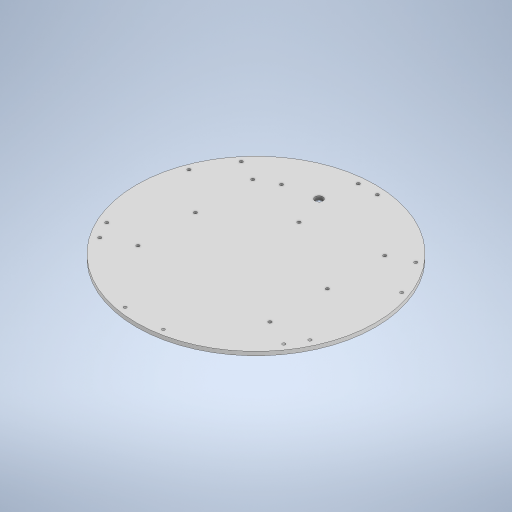
# Autodesk Inventor part: 中間台1
Saved by Autodesk Inventor 2023 (Build 270158000, 158)
## iProperties
Created: 2022-12-03
Part Number: 中間台1
Material: 一般
Document SubType Name: Modeling
Designer: RiSA
Density: 1 g/cm^3
Appearance: 既定
Author: RiSA
Autodesk Inventor part; units mm, degrees
ref_plane "YZ Plane" through (0, 0, 0) normal (1, 0, 0) x (0, 1, 0)
ref_plane "XZ Plane" through (0, 0, 0) normal (0, 1, 0) x (-1, 0, 0)
ref_plane "XY Plane" through (0, 0, 0) normal (0, 0, 1) x (1, 0, 0)
sketch "スケッチ1" plane through (0, 0, 0) normal (0, 1, 0) x (-1, 0, 0)
  circle A0 centre (0, 0) radius 125
  dimension "d0" = 250
  constraints: 1 centre point, 1 coincident
  measures "d0" diameter of A0
extrude "押し出し1" add sketch "スケッチ1" along normal blind 4
sketch "スケッチ2" plane through (0, 4, 0) normal (0, 1, 0) x (1, 0, 0)
  line L0 (75, -84.411) -> (-75, -84.411)
  line L1 (-75, -84.411) -> (-75, 95.589)
  line L2 (-75, 95.589) -> (75, 95.589)
  line L3 (75, 95.589) -> (75, -84.411)
  line L4 (75, -84.411) -> (-75, 95.589) construction
  line L5 (-75, -84.411) -> (75, 95.589) construction
  circle A0 centre (0, 0) radius 121.5
  line L6 (0, 0) -> (0, -125) construction
  circle A1 centre (0, 0) radius 125 projected
  line L7 (0, 0) -> (108.2532, 62.5) construction
  line L8 (0, 0) -> (-108.2532, 62.5) construction
  circle A2 centre (-16.75, 82.589) radius 4.1
  point P0 (0, 5.589)
  dimension "d3" = 150
  dimension "d4" = 180
  dimension "d5" = 243
  dimension "d8" = 360
  dimension "d12" = 16.75
  dimension "d13" = 13
  dimension "d14" = 8.2
  constraints: 18 end point, 2 centre point, 2 coincident, 2 midpoint, 2 parallel, 2 point on circle, 1 horizontal, 1 perpendicular, 1 vertical, 1 vertical alignment, 11 other
  measures "d3" distance of L1.end L2.end
  measures "d4" distance of L0.end L1.end
  measures "d5" diameter of A0
  measures "d12" horizontal distance of point (0, 0) point (-16.75, 82.589)
  measures "d13" distance from line of L2 point (-16.75, 82.589)
  measures "d14" diameter of A2
extrude "押し出し2" cut sketch "スケッチ2" against normal blind 4 contours A2
sketch "スケッチ4" plane through (0, 4, 0) normal (0, 1, 0) x (1, 0, 0)
  circle A0 centre (0, 0) radius 121.5
  line L0 (75, -84.411) -> (-75, -84.411)
  line L1 (-75, -84.411) -> (-75, 95.589)
  line L2 (-75, 95.589) -> (75, 95.589)
  line L3 (75, 95.589) -> (75, -84.411)
  line L4 (75, -84.411) -> (-75, 95.589) construction
  line L5 (-75, -84.411) -> (75, 95.589) construction
  line L6 (0, 0) -> (0, -29.9183)
  point P0 (0, 5.589)
  point P1 (69, -54.411)
  point P2 (69, 5.589)
  point P3 (69, 65.589)
  point P4 (-69, -54.411)
  point P5 (-69, 5.589)
  point P6 (-69, 65.589)
  dimension "d17" = 243
  dimension "d18" = 150
  dimension "d19" = 180
  dimension "d20" = 30
  dimension "d21" = 6
  dimension "d22" = 60
  dimension "d23" = 60
  constraints: 14 end point, 3 symmetric about line, 2 midpoint, 2 parallel, 2 point on circle, 1 centre point, 1 coincident, 1 horizontal, 1 perpendicular, 1 vertical
  measures "d17" diameter of A0
  measures "d18" distance of L1.end L2.end
  measures "d19" distance of L0.end L1.end
  measures "d20" distance from line of L0 point (69, -54.411)
  measures "d21" distance from line of L3 point (69, -54.411)
  measures "d22" distance of point (69, -54.411) point (69, 5.589)
  measures "d23" distance of point (69, 5.589) point (69, 65.589)
hole "穴1" at (69, 4, 54.411) at (69, 4, -5.589) at (69, 4, -65.589) at (-69, 4, -65.589) at (-69, 4, -5.589) at (-69, 4, 54.411) direction (0, -1, 0) diameter 3.2 end through all
sketch "スケッチ5" plane through (0, 4, 0) normal (0, 1, 0) x (1, 0, 0)
  point P0 (0, 0)
  point P1 (0, -116.86)
  point P2 (20, -116.86)
  point P3 (-20, -116.86)
  point P4 (111.2037, 41.1095)
  point P5 (91.2037, 75.7505)
  point P6 (101.2037, 58.43)
  point P7 (-91.2037, 75.7505)
  point P8 (-111.2037, 41.1095)
  point P9 (-101.2037, 58.43)
  dimension "d31" = 116.86
  dimension "d32" = 20
  dimension "d33" = 20
  dimension "d36" = 360
  constraints: 10 other
  measures "d31" distance of point (0, 0) point (0, -116.86)
  measures "d32" distance of point (0, -116.86) point (20, -116.86)
  measures "d33" distance of point (-20, -116.86) point (0, -116.86)
hole "穴2" at (20, 4, 116.86) at (-20, 4, 116.86) at (111.2037, 4, -41.1095) at (91.2037, 4, -75.7505) at (-91.2037, 4, -75.7505) at (-111.2037, 4, -41.1095) direction (0, -1, 0) diameter 3.2 depth 10
sketch "スケッチ6" plane through (0, 4, 0) normal (0, 1, 0) x (1, 0, 0)
  point P0 (0, 0)
  point P1 (0, 116.86)
  point P2 (-10, 116.86)
  point P3 (10, 116.86)
  point P4 (-106.2037, -49.7697)
  point P5 (-96.2037, -67.0903)
  point P6 (-101.2037, -58.43)
  point P7 (96.2037, -67.0903)
  point P8 (106.2037, -49.7697)
  point P9 (101.2037, -58.43)
  dimension "d45" = 116.86
  dimension "d46" = 10
  dimension "d47" = 10
  dimension "d50" = 360
  constraints: 10 other
  measures "d45" distance of point (0, 0) point (0, 116.86)
  measures "d46" distance of point (0, 116.86) point (-10, 116.86)
  measures "d47" distance of point (0, 116.86) point (10, 116.86)
hole "穴3" at (-10, 4, -116.86) at (10, 4, -116.86) at (-106.2037, 4, 49.7697) at (-96.2037, 4, 67.0903) at (96.2037, 4, 67.0903) at (106.2037, 4, 49.7697) direction (0, -1, 0) diameter 3.2 depth 10
sketch "スケッチ7" plane through (0, 4, 0) normal (0, 1, 0) x (1, 0, 0)
  circle A0 centre (-16.75, 82.589) radius 4.1 projected
  line L0 (-16.75, 82.589) -> (-27.75, 63.5364) construction
  line L1 (-16.75, 82.589) -> (5.25, 82.589) construction
  line L2 (-27.75, 63.5364) -> (-49.4006, 76.0364)
  line L3 (-49.4006, 76.0364) -> (-6.0994, 51.0364) construction
  point P0 (0, 0)
  dimension "d59" = 22
  dimension "d60" = 120
  dimension "d61" = 25
  dimension "d62" = 50
  constraints: 8 end point, 2 coincident, 1 equal length, 1 horizontal, 1 point on line
  measures "d59" distance of L0.start L0.end
  measures "d60" angle of L0 L1
  measures "d61" distance of L0.end L2.end
  measures "d62" distance of L2.end L3.end
hole "穴4" at (-49.4006, 4, -76.0364) at (-6.0994, 4, -51.0364) direction (0, -1, 0) diameter 3.2 depth 10
